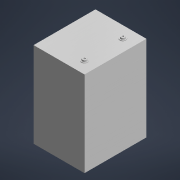
# Autodesk Inventor part: Batería
Saved by Autodesk Inventor 2022 (Build 260153000, 153)
## iProperties
Part Number: Batería
Material: Genérico
Document SubType Name: Modelado
Designer: seb_0
Appearance: PVC - Blanco
Mass: 16000 g
Surface Area: 2696.66 cm^2
Volume: 9174.6 cm^3
Density: 1.74395 g/cm^3
Author: seb_0
Autodesk Inventor part; units mm, degrees
ref_plane "Plano YZ" through (0, 0, 0) normal (1, 0, 0) x (0, 1, 0)
ref_plane "Plano XZ" through (0, 0, 0) normal (0, 1, 0) x (-1, 0, 0)
ref_plane "Plano XY" through (0, 0, 0) normal (0, 0, 1) x (1, 0, 0)
sketch "Boceto1" plane through (0, 0, 0) normal (0, 1, 0) x (-1, 0, 0)
  line L0 (0, 0) -> (165.1, 0)
  line L1 (165.1, 0) -> (165.1, -200.66)
  line L2 (165.1, -200.66) -> (0, -200.66)
  line L3 (0, -200.66) -> (0, 0)
  dimension "d0" = 200.66
  dimension "d1" = 165.1
  constraints: 8 end point, 2 parallel, 1 horizontal, 1 perpendicular
  measures "d0" distance of L2.end L0.start
  measures "d1" distance of L0.start L0.end
extrude "Extrusión1" add sketch "Boceto1" along normal blind 276.86
sketch "Boceto2" plane through (0, 276.86, 0) normal (0, 1, 0) x (1, 0, 0)
  circle A0 centre (-38.1, 38.1) radius 10
  circle A1 centre (-38.1, 162.56) radius 10
  line L0 (0, 0) -> (0, 200.66) projected
  line L1 (-165.1, 0) -> (0, 0) projected
  dimension "d4" = 20
  dimension "d6" = 124.46
  dimension "d7" = 38.1
  dimension "d8" = 38.1
  dimension "d9" = 38.1
  constraints: 2 centre point, 1 equal radius
  measures "d4" diameter of A0
  measures "d6" distance of A1.centre A0.centre
  measures "d7" distance from line of L0 A0.centre
  measures "d8" distance from line of L0 A1.centre
  measures "d9" distance from line of L1 A0.centre
extrude "Extrusión2" add sketch "Boceto2" along normal blind 7
sketch "Boceto3" plane through (-38.1, 283.86, -38.1) normal (0, 1, 0) x (1, 0, 0)
  circle A0 centre (0, 0) radius 10 projected
  circle A1 centre (0, 124.46) radius 10 projected
  circle A2 centre (0, 124.46) radius 3
  circle A3 centre (0, 0) radius 3
  circle A4 centre (0, 0) radius 7
  circle A5 centre (0, 124.46) radius 7
  point P0 (38.1, -38.1)
  dimension "d12" = 6
  dimension "d13" = 6
  dimension "d16" = 14
  dimension "d17" = 14
  constraints: 4 centre point, 4 coincident
  measures "d12" diameter of A2
  measures "d13" diameter of A3
  measures "d16" diameter of A4
  measures "d17" diameter of A5
extrude "Extrusión3" cut sketch "Boceto3" against normal blind 5
